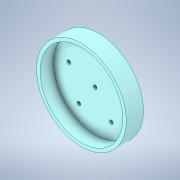
# Autodesk Inventor part: Wheel
Saved by Autodesk Inventor 2020.1 (Build 241239000, 239)
## iProperties
Created: 2019-11-14
Part Number: Wheel
Material: Generic
Document SubType Name: Modeling
Designer: Ali
Density: 1 g/cm^3
Appearance: Default
Author: Ali
Autodesk Inventor part; units mm, degrees
ref_plane "YZ Plane" through (0, 0, 0) normal (1, 0, 0) x (0, 1, 0)
ref_plane "XZ Plane" through (0, 0, 0) normal (0, 1, 0) x (-1, 0, 0)
ref_plane "XY Plane" through (0, 0, 0) normal (0, 0, 1) x (1, 0, 0)
sketch "Sketch1" plane through (0, 0, 0) normal (0, 0, 1) x (1, 0, 0)
  line L0 (0, 0) -> (50.8, 0) construction
  line L1 (0, 82.55) -> (0, 76.2)
  line L2 (0, 76.2) -> (50.8, 76.2)
  line L3 (50.8, 76.2) -> (50.8, 82.55)
  line L4 (50.8, 82.55) -> (0, 82.55)
  dimension "d1" = 50.8
  dimension "d7" = 76.2
  dimension "d8" = 6.35
  constraints: 10 end point, 2 perpendicular, 2 vertical, 1 horizontal
  measures "d1" distance of L1.end L2.end
  measures "d7" distance between parallel lines of L0 L2
  measures "d8" distance of L1.start L1.end
revolve "Revolution1" add sketch "Sketch1" angle 360 about axis through (0, 0, 0) along (1, 0, 0)
sketch "Sketch2" plane through (50.8, 0, 0) normal (1, 0, 0) x (0, 0, -1)
  circle A0 centre (0, 0) radius 82.55 projected
  circle A1 centre (0, 0) radius 76.2 projected
extrude "Extrusion1" add sketch "Sketch2" along normal blind 6.35 contours A0 | A1
sketch "Sketch3" plane through (50.8, 0, 0) normal (-1, 0, 0) x (0, 0, 1)
  point P0 (0, 0)
  point P1 (0, 50.8)
  point P2 (0, 0)
  dimension "d9" = 50.8
  constraints: 1 coincident
  measures "d9" distance of point (0, 0) point (0, 50.8)
hole "Hole1" at (50.8, 50.8, 0) at (50.8, 0, 0) direction (1, 0, 0) diameter 6.858 end through all
pattern_circular "Circular Pattern1" count 5 over 360 about axis through (25.4, 0, 0) along (1, 0, 0) of "Hole1"
ref_plane "Work Plane2" through (25.4, 0, 0) normal (-1, 0, 0) x (0, 0, 1)
sketch "Sketch7" plane through (25.4, 0, 0) normal (-1, 0, 0) x (0, 0, 1)
  circle A0 centre (0, 0) radius 76.2 projected
  circle A1 centre (0, 0) radius 82.55 projected
extrude "Extrusion4" cut sketch "Sketch7" along normal through all
equation "\"d1\" = wheelDepth"
equation "\"d7\" = wheelR"
equation "\"d8\" = wheelThickness"
equation "\"d9\" = farFromCenter"
equation "\"d10\" = smallHoles"
equation "\"gearShaft\" = 6.35"
equation "\"largeGear\" = 38.1"
equation "\"smallGear\" = 12.7"
equation "\"wheelR\" = 76.2"
equation "\"wheelThickness\" = 6.35"
equation "\"wheelDepth\" = 50.8"
equation "\"mainHole\" = 6.858"
equation "\"smallHoles\" = 6.858"
equation "\"farFromCenter\" = 50.8"
equation "\"smallGearLength\" = 50.8"
equation "\"mainGearLength\" = 76.2"
equation "\"gearThickness\" = 6.35"
equation "\"mainGear\" = 38.1"
equation "\"swivelBaseDiameter\" = 19.05"
equation "\"swivelLegExtentions\" = 19.05"
equation "\"swivelLegLength\" = 49.13565"
equation "\"swivelLegThickness\" = 19.05"
equation "\"d41\" = 0.5 * wheelDepth"
body "Solid1"
